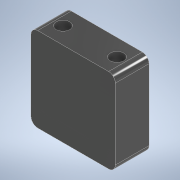
# Autodesk Inventor part: pendulum_mass
Saved by Autodesk Inventor 2021 (Build 250183000, 183)
## iProperties
Created: 2022-06-20
Part Number: pendulum_mass
Material: ABS Plastic
Document SubType Name: Modeling
Designer: lenna
Density: 1.06 g/cm^3
Appearance: Dark Gray
Author: lenna
Autodesk Inventor part; units mm, degrees
ref_plane "YZ Plane" through (0, 0, 0) normal (1, 0, 0) x (0, 1, 0)
ref_plane "XZ Plane" through (0, 0, 0) normal (0, 1, 0) x (-1, 0, 0)
ref_plane "XY Plane" through (0, 0, 0) normal (0, 0, 1) x (1, 0, 0)
sketch "Sketch1" plane through (0, 0, 0) normal (0, 0, 1) x (1, 0, 0)
  line L0 (-12.5, 12.5) -> (12.5, 12.5)
  line L1 (12.5, 12.5) -> (12.5, -12.5)
  line L2 (12.5, -12.5) -> (-12.5, -12.5)
  line L3 (-12.5, -12.5) -> (-12.5, 12.5)
  point P0 (0, 0)
  dimension "d2" = 25
  dimension "d3" = 12.5
  dimension "d4" = 25
  dimension "d5" = 12.5
  constraints: 8 end point, 2 parallel, 1 horizontal, 1 perpendicular
  measures "d2" distance between parallel lines of L1 L3
  measures "d3" distance from line of point (0, 0) L3
  measures "d4" distance between parallel lines of L2 L0
  measures "d5" distance from line of point (0, 0) L0
extrude "Extrusion1" add sketch "Sketch1" along normal blind 10
sketch "Sketch2" plane through (-12.5, 12.5, 0) normal (0, 1, 0) x (1, 0, 0)
  line L0 (25, -10) -> (0, -10) projected
  line L1 (25, 0) -> (0, 0) projected
  line L2 (0, 0) -> (0, -10) projected
  point P0 (12.5, 0)
  point P1 (4.5, -5)
  dimension "d8" = 10
  dimension "d9" = 5
  dimension "d18" = 8
  measures "d8" distance between parallel lines of L0 L1
  measures "d9" distance from line of L1 point (4.5, -5)
  measures "d18" horizontal distance of point (12.5, 0) point (4.5, -5)
hole "Hole1" at (-8, 12.5, 5) direction (0, -1, 0) diameter 4 depth 25
mirror "Mirror1" about plane through (0, 0, 0) normal (1, 0, 0) of "Hole1"
sketch "Sketch3" plane through (-12.5, -12.5, 0) normal (0, -1, 0) x (1, 0, 0)
  line L0 (0, 0) -> (25, 0) projected
  line L1 (0, 10) -> (25, 10) projected
  line L2 (0, 0) -> (0, 10) projected
  line L3 (25, 0) -> (25, 10) projected
  point P0 (12.5, 0)
  point P1 (12.5, 5)
  dimension "d19" = 10
  dimension "d20" = 25
  dimension "d21" = 12.5
  dimension "d22" = 5
  measures "d19" distance between parallel lines of L0 L1
  measures "d20" distance between parallel lines of L2 L3
  measures "d21" distance from line of L2 point (12.5, 5)
  measures "d22" distance from line of L0 point (12.5, 5)
hole "Hole2" at (0, -12.5, 5) direction (0, 1, 0) diameter 8 depth 20
chamfer "Chamfer1" distance 0.5 angle 45 1 edges at (0, -12.5, 9)
fillet "Fillet1" radius 2 4 edges at (-12.5, -12.5, 5) (-12.5, 12.5, 5) (12.5, 12.5, 5) (12.5, -12.5, 5)
equation "\"d3\" = 0.5 * d2"
equation "\"d5\" = 0.5 * d4"
equation "\"d9\" = 0.5 * d8"
equation "\"d21\" = 0.5 * d20"
equation "\"d22\" = 0.5 * d19"
body "Solid1"
